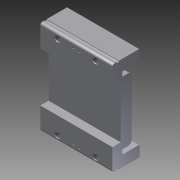
# Autodesk Inventor part: KR55-A-Slider Spacer
Saved by Autodesk Inventor 2011 SP1 (Build 150282100, 282)
## iProperties
Created: 2013-10-23
Part Number: KR55-A-Slider Spacer
Catalog Web Link: www.cadenas.de
Description: LM Guide Actuator - Slider Spacer-KR
Vendor: THK
Document SubType Name: Modeling
Designer: PARTuser1
Manufacturer: THK
Density: 1 g/cm^3
Category: PARTsolutions
Company: THK
Title: KR55-A-Slider Spacer
Author: Cadenas PARTsolutions
Comments: KR
PSOL_IDENT_0: {$CADENAS_DATA\23d-libs\thk\lm_guide_actuator\type_kr\parts\lm_g_a_kr_slider_spacer.prj},214 {VTYP=3
PSOL_IDENT_1: D},{NB=KR55-A-Slider Spacer},{LINA=KR55-A-Slider Spacer},{NN=LM Guide Actuator - Slider Spacer},{DAT
PSOL_IDENT_2: E=17.05.2010 06:34:46},{GEOMDATE=07.11.2007 11:59:00},{VERSION=},{LINEID=80},{LINESUBID=-1},{WBVAR=T
PSOL_IDENT_3: YPE1}  {NB=KR55-A-Slider Spacer},{LINA=KR55-A-Slider Spacer},{KT=DUMMY},{ORDER=KR55},{XTYPE2=8.000},
PSOL_IDENT_4: {TYPE1=A},{TYPE2='A','B'},{XTYPE=1}
CNS_NT: KR
CNS_NB: KR55-A-Slider Spacer
CNS_NBSYN: $ORDER.-$TYPE1.-Slider Spacer
CNS_LINA: KR55-A-Slider Spacer
CNS_ORDER: KR55
CNS_XTYPE2: 8.000
CNS_TYPE1: A
CNS_TYPE2: 'A','B'
CNS_XTYPE: 1.000
SUPPLIER: THK
ARTICLENO: KR55-A-Slider Spacer
BOMINFO: KR55-A-Slider Spacer
CREATOR: CADENAS GmbH
Autodesk Inventor part; units mm, degrees
sketch "Sketch_1" plane through (0, 0, 0) normal (1, 0, 0) x (0, 1, 0)
  line L0 (24, 62) -> (-2.5, 62)
  arc A0 (-5.5, 62) -> (-2.5, 62) centre (-4, 62) ccw
  line L1 (-5.5, 62) -> (-8, 62)
  arc A1 (-8, 62) -> (-11, 59) centre (-8, 59) ccw
  line L2 (-11, 59) -> (-11, 32.5)
  line L3 (-11, 32.5) -> (0, 32.5)
  line L4 (0, 32.5) -> (0, -32.5)
  line L5 (0, -32.5) -> (-11, -32.5)
  line L6 (-11, -32.5) -> (-11, -59)
  arc A2 (-11, -59) -> (-8, -62) centre (-8, -59) ccw
  line L7 (-8, -62) -> (-5.5, -62)
  arc A3 (-2.5, -62) -> (-5.5, -62) centre (-4, -62) ccw
  line L8 (-2.5, -62) -> (24, -62)
  arc A4 (24, -62) -> (25, -61) centre (24, -61) ccw
  line L9 (25, -61) -> (25, -48.5)
  arc A5 (25, -48.5) -> (24, -47.5) centre (24, -48.5) ccw
  line L10 (24, -47.5) -> (3, -47.5)
  arc A6 (2, -46.5) -> (3, -47.5) centre (3, -46.5) ccw
  line L11 (2, -46.5) -> (2, -42.5)
  arc A7 (3, -41.5) -> (2, -42.5) centre (3, -42.5) ccw
  line L12 (3, -41.5) -> (9.5, -41.5)
  arc A8 (9.5, -41.5) -> (14.5, -36.5) centre (9.5, -36.5) ccw
  line L13 (14.5, -36.5) -> (14.5, 36.5)
  arc A9 (14.5, 36.5) -> (9.5, 41.5) centre (9.5, 36.5) ccw
  line L14 (9.5, 41.5) -> (3, 41.5)
  arc A10 (2, 42.5) -> (3, 41.5) centre (3, 42.5) ccw
  line L15 (2, 42.5) -> (2, 46.5)
  arc A11 (3, 47.5) -> (2, 46.5) centre (3, 46.5) ccw
  line L16 (3, 47.5) -> (24, 47.5)
  arc A12 (24, 47.5) -> (25, 48.5) centre (24, 48.5) ccw
  line L17 (25, 48.5) -> (25, 61)
  arc A13 (25, 61) -> (24, 62) centre (24, 61) ccw
  constraints: 36 end point, 28 point on circle, 14 centre point
extrude "Extrusion1" add sketch "Sketch_1" along normal mid plane 95.2
sketch "Sketch2" plane through (-47.6, -11, 59) normal (0, -1, 0) x (1, 0, 0)
  point P0 (22.6, -4)
hole "Drilling 1" at (-25, -11, 55) direction (0, 1, 0) diameter 6.647 depth 36 countersink diameter 8 countersink angle 90 thread size "M8x1.25" class "6H" standard "ISO Metric profile"
pattern_linear "Rectangular Pattern1" count 2 spacing 50 along (1, 0, 0) count 2 spacing 110 along (0, 0, -1) of "Drilling 1"
sketch "Sketch3" plane through (-47.6, -11, 32.5) normal (0, -1, 0) x (1, 0, 0)
  point P0 (43.6, 22.5)
hole "Drilling 2" at (-4, -11, 55) direction (0, 1, 0) diameter 2.459 depth 7 tip angle 140 countersink diameter 3 countersink angle 90 thread size "M3x0.5" class "6H" standard "ISO Metric profile"
pattern_linear "Rectangular Pattern2" count 2 spacing 8 along (1, 0, 0) count 2 spacing 110 along (0, 0, -1) of "Drilling 2"
ref_plane "slider_spacer_sensor_dog_XY" through (0, -11, 55) normal (0, 1, 0) x (1, 0, 0)
ref_plane "slider_spacer_sensor_dog_YZ" through (0, -11, 55) normal (1, 0, 0) x (0, 0, -1)
ref_plane "slider_spacer_sensor_dog_ZX" through (0, -11, 55) normal (0, 0, -1) x (0, 1, 0)
ref_plane "slider_spacer_slider_XY" through (0, 0, 0) normal (0, 1, 0) x (1, 0, 0)
ref_plane "slider_spacer_slider_YZ" through (0, 0, 0) normal (1, 0, 0) x (0, 0, -1)
ref_plane "slider_spacer_slider_ZX" through (0, 0, 0) normal (0, 0, -1) x (0, 1, 0)
body "Solid1"
